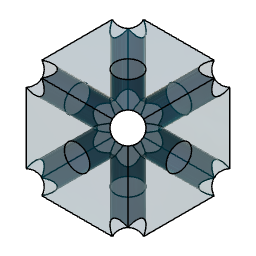
0.25 cm lattice v2 (Autodesk Fusion 360 design; units mm, degrees)
Autodesk Fusion 360 part; units mm, degrees
sketch "Sketch1" plane through (0, 0, 0) normal (0, 0, 1) x (1, 0, 0)
  circle A0 centre (0, 0) radius 1.25
  line L0 (5, -5) -> (-5, -5)
  line L1 (-5, -5) -> (-5, 5)
  line L2 (-5, 5) -> (5, 5)
  line L3 (5, 5) -> (5, -5)
  line L4 (5, -5) -> (-5, 5) construction
  line L5 (-5, -5) -> (5, 5) construction
  line L6 (0, -5) -> (0, 5) construction
  line L7 (5, 0) -> (-5, 0) construction
  dimension "d1" = 2.5
  dimension "d3" = 10
  dimension "d4" = 10
  constraint coincident A0.centre origin
  constraint perpendicular L0 L1
  constraint parallel L0 L2
  constraint parallel L1 L3
  constraint horizontal L0
  constraint coincident L4 A0.centre
  constraint coincident L5 A0.centre
  constraint midpoint L0 L6.start
  constraint midpoint L2 L6.end
  constraint midpoint L3 L7.start
  constraint perpendicular L3 L7
  measures "d1" diameter of A0
  measures "d3" distance of L0.end L1.end
  measures "d4" distance of L1.end L2.end
ref_plane "WorkPlane1" through (0, -5, 0) normal (0, 1, 0) x (-1, 0, 0)
sketch "Sketch2" plane through (0, -5, 0) normal (0, 1, 0) x (1, 0, 0)
  line L0 (-5, 0) -> (5, 0)
  line L1 (5, 0) -> (5, -10)
  line L2 (5, -10) -> (-5, -10)
  line L3 (-5, -10) -> (-5, 0)
  line L4 (0, 0) -> (0, -10) construction
  circle A0 centre (0, -5) radius 1.25
  point P0 (5, 0)
  point P1 (-5, 0)
  point P2 (5, 0)
  dimension "d6" = 10
  dimension "d8" = 2.5
  constraint horizontal L0
  constraint vertical L1
  constraint horizontal L2
  constraint vertical L3
  constraint coincident P1 L0.start
  constraint coincident L4.start origin
  constraint midpoint L2 L4.end
  constraint perpendicular L2 L4
  constraint midpoint L4 A0.centre
  measures "d6" distance of P1 L2.end
  measures "d8" diameter of A0
ref_plane "WorkPlane2" through (-5, 0, 0) normal (1, 0, 0) x (0, 1, 0)
sketch "Sketch3" plane through (-5, 0, 0) normal (1, 0, 0) x (0, 1, 0)
  line L0 (5, 0) -> (-5, 0)
  line L1 (-5, 0) -> (-5, 10)
  line L2 (-5, 10) -> (5, 10)
  line L3 (5, 10) -> (5, 0)
  line L4 (0, 0) -> (0, 10) construction
  circle A0 centre (0, 5) radius 1.25
  point P0 (-5, 0)
  point P1 (-5, 10)
  point P2 (5, 0)
  dimension "d10" = 2.5
  constraint horizontal L0
  constraint vertical L1
  constraint horizontal L2
  constraint vertical L3
  constraint coincident P1 L1.end
  constraint coincident P2 L0.start
  constraint coincident L4.start origin
  constraint midpoint L2 L4.end
  constraint midpoint L4 A0.centre
  measures "d10" diameter of A0
ref_plane "WorkPlane3" through (0, 5, 0) normal (0, -1, 0) x (1, 0, 0)
sketch "Sketch4" plane through (0, 5, 0) normal (0, -1, 0) x (1, 0, 0)
  line L0 (5, 0) -> (5, 10)
  line L1 (5, 10) -> (-5, 10)
  circle A0 centre (0, 5) radius 1.25
  line L2 (-5, 0) -> (-5, 10)
  line L3 (-5, 0) -> (5, 0)
ref_plane "WorkPlane4" through (5, 0, 0) normal (-1, 0, 0) x (0, -1, 0)
sketch "Sketch5" plane through (5, 0, 0) normal (-1, 0, 0) x (0, 1, 0)
  line L0 (-5, -10) -> (-5, 0)
  line L1 (-5, -10) -> (5, -10)
  circle A0 centre (0, -5) radius 1.25
  line L2 (5, 0) -> (-5, 0)
  line L3 (5, -10) -> (5, 0)
ref_plane "WorkPlane5" through (0, -5, 10) normal (0, 0, 1) x (-1, 0, 0)
sketch "Sketch6" plane through (0, -5, 10) normal (0, 0, 1) x (1, 0, 0)
  line L0 (-5, 0) -> (5, 0)
  circle A0 centre (0, 5) radius 1.25
  line L1 (-5, 10) -> (5, 10)
  line L2 (-5, 0) -> (-5, 10)
  line L3 (5, 10) -> (5, 0)
ref_plane "WorkPlane6" through (-5, 5, 0) normal (0.57735, -0.57735, -0.57735) x (0.707107, 0.707107, 0)
ref_plane "WorkPlane7" through (-8.3333, 8.3333, 3.3333) normal (0.57735, -0.57735, -0.57735) x (0.707107, 0.707107, 0)
sketch "Sketch7" plane through (-8.3333, 8.3333, 3.3333) normal (0.57735, -0.57735, -0.57735) x (0.707107, 0.707107, 0)
  circle A0 centre (0, 8.165) radius 1.25
  point P0 (0, 8.165)
  point P1 (0, 8.165)
  point P2 (0, 8.165)
  dimension "d25" = 2.5
  constraint coincident P1 P0
  measures "d25" diameter of A0
ref_plane "WorkPlane8" through (-5, -5, 0) normal (0.57735, 0.57735, -0.57735) x (-0.707107, 0.707107, 0)
ref_plane "WorkPlane9" through (-8.3333, -8.3333, 3.3333) normal (0.57735, 0.57735, -0.57735) x (-0.707107, 0.707107, 0)
sketch "Sketch8" plane through (-8.3333, -8.3333, 3.3333) normal (0.57735, 0.57735, -0.57735) x (-0.707107, 0.707107, 0)
  circle A0 centre (0, 8.165) radius 1.25
  point P0 (0, 8.165)
  point P1 (0, 8.165)
  point P2 (0, 8.165)
  dimension "d24" = 2.5
  constraint coincident P2 P0
  measures "d24" diameter of A0
ref_plane "WorkPlane10" through (5, -5, 0) normal (-0.57735, 0.57735, -0.57735) x (-0.707107, -0.707107, 0)
ref_plane "WorkPlane11" through (8.3333, -8.3333, 3.3333) normal (-0.57735, 0.57735, -0.57735) x (-0.707107, -0.707107, 0)
sketch "Sketch9" plane through (8.3333, -8.3333, 3.3333) normal (-0.57735, 0.57735, -0.57735) x (-0.707107, -0.707107, 0)
  circle A0 centre (0, 8.165) radius 1.25
  point P0 (0, 8.165)
  point P1 (0, 8.165)
  point P2 (0, 8.165)
  dimension "d23" = 2.5
  constraint coincident P2 P0
  measures "d23" diameter of A0
ref_plane "WorkPlane12" through (5, 5, 0) normal (-0.57735, -0.57735, -0.57735) x (0.707107, -0.707107, 0)
ref_plane "WorkPlane13" through (8.3333, 8.3333, 3.3333) normal (-0.57735, -0.57735, -0.57735) x (0.707107, -0.707107, 0)
sketch "Sketch10" plane through (8.3333, 8.3333, 3.3333) normal (-0.57735, -0.57735, -0.57735) x (0.707107, -0.707107, 0)
  circle A0 centre (0, 8.165) radius 1.25
  point P0 (0, 8.165)
  point P1 (0, 8.165)
  point P2 (0, 8.165)
  dimension "d22" = 2.5
  constraint coincident P2 P1
  measures "d22" diameter of A0
extrude "Extrude1" add sketch "Sketch1" along normal up to surface (10 mm away) contours A0 | L0 L1 L2 L3
extrude "Extrude2" cut sketch "Sketch3" along normal through all contours A0
extrude "Extrude3" cut sketch "Sketch2" along normal through all contours A0
extrude "Extrude4" cut sketch "Sketch1" along normal through all contours A0
extrude "Extrude5" cut sketch "Sketch10" along normal through all
extrude "Extrude6" cut sketch "Sketch7" along normal through all
extrude "Extrude7" cut sketch "Sketch8" along normal through all
extrude "Extrude8" cut sketch "Sketch9" along normal through all
equation "d1 = TubeDiamter"
equation "TubeDiamter = 2.5 mm"
equation "d3 = CubeSize"
equation "d4 = CubeSize"
equation "d6 = CubeSize"
equation "CubeSize = 10 mm"
equation "d8 = TubeDiamter"
equation "d10 = TubeDiamter"
equation "d22 = TubeDiamter"
equation "d23 = TubeDiamter"
equation "d24 = TubeDiamter"
equation "d25 = TubeDiamter"
